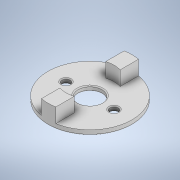
# Autodesk Inventor part: tensioner_servo
Saved by Autodesk Inventor 2022 (Build 260153000, 153)
## iProperties
Created: 2022-02-27
Part Number: tensioner_servo
Material: Generic
Document SubType Name: Modeling
Designer: Frey
Density: 1 g/cm^3
Appearance: Default
Author: Frey
Autodesk Inventor part; units mm, degrees
ref_plane "YZ Plane" through (0, 0, 0) normal (1, 0, 0) x (0, 1, 0)
ref_plane "XZ Plane" through (0, 0, 0) normal (0, 1, 0) x (-1, 0, 0)
ref_plane "XY Plane" through (0, 0, 0) normal (0, 0, 1) x (1, 0, 0)
sketch "Sketch1" plane through (0, 0, 0) normal (0, 1, 0) x (-1, 0, 0)
  circle A0 centre (0, 0) radius 17.5
  dimension "d0" = 35
  constraints: 1 centre point, 1 coincident
  measures "d0" diameter of A0
extrude "Extrusion1" add sketch "Sketch1" along normal blind 2
sketch "Sketch2" plane through (0, 2, 0) normal (0, 1, 0) x (1, 0, 0)
  arc A0 (-3, -9.5394) -> (3, -9.5394) centre (0, 0) ccw
  line L0 (-3, -17.2409) -> (-3, -9.5394)
  line L1 (3, -17.2409) -> (3, -9.5394)
  line L2 (-3, 9.5394) -> (-3, 17.2409)
  circle A1 centre (0, 0) radius 17.5 projected
  line L3 (3, 9.5394) -> (3, 17.2409)
  arc A2 (-3, 9.5394) -> (-3, -9.5394) centre (0, 0) ccw construction
  arc A3 (3, -9.5394) -> (3, 9.5394) centre (0, 0) ccw construction
  arc A4 (3, 9.5394) -> (-3, 9.5394) centre (0, 0) ccw
  dimension "d3" = 20
  dimension "d4" = 6
  dimension "d5" = 3
  constraints: 13 point on circle, 8 end point, 4 centre point, 4 point on line, 1 coincident, 1 parallel, 1 vertical
  measures "d3" diameter of A0
  measures "d4" distance between parallel lines of L1 L0
  measures "d5" distance from line of point (0, 0) L0
extrude "Extrusion2" add sketch "Sketch2" along normal blind 6 contours A0 L1 A1 L0 | A1 L3 A4 L2
sketch "Sketch3" plane through (0, 2, 0) normal (0, 1, 0) x (1, 0, 0)
  circle A0 centre (-10, 0) radius 1.75
  circle A1 centre (10, 0) radius 1.75
  point P0 (0, 0)
  dimension "d8" = 3.5
  dimension "d9" = 20
  dimension "d10" = 10
  dimension "d11" = 3.5
  constraints: 2 centre point, 2 horizontal alignment
  measures "d8" diameter of A0
  measures "d9" distance of A1.centre A0.centre
  measures "d10" distance of point (0, 0) A0.centre
  measures "d11" diameter of A1
extrude "Extrusion3" cut sketch "Sketch3" against normal up to surface (2 mm away)
sketch "Sketch4" plane through (0, 0, 0) normal (0, -1, 0) x (1, 0, 0)
  circle A0 centre (0, 0) radius 5
  dimension "d14" = 10
  constraints: 1 centre point, 1 coincident
  measures "d14" diameter of A0
extrude "Extrusion4" cut sketch "Sketch4" against normal up to surface (2 mm away)
fillet "Fillet1" radius 0.4 7 edges at (-5, 0, 0) (-5, 2, 0) (17.5, 0, 0) (-11.75, 2, 0) (8.25, 2, 0) (8.25, 0, 0) (-11.75, 0, 0)
body "Solid1"
